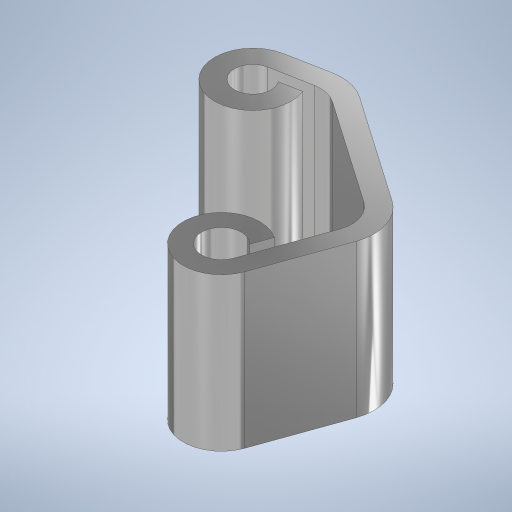
# Autodesk Inventor part: Linkage for inset hinge
Saved by Autodesk Inventor 2024 (Build 280153000, 153)
## iProperties
Created: 2008-03-26
Part Number: Linkage for inset hinge
Document SubType Name: Modeling
Designer: G.K.
Material: Steel
Description: Linkage for inset hinge
Authority: Design by UAB Čeli APS
Mass: 4.02681 g
Surface Area: 9.41342 cm^2
Volume: 0.512969 cm^3
Density: 7.85 g/cm^3
Appearance: Chrome - Polished
Mase: 0.00402681
Autodesk Inventor part; units mm, degrees
ref_plane "YZ Plane" through (0, 0, 0) normal (1, 0, 0) x (0, 1, 0)
ref_plane "XZ Plane" through (0, 0, 0) normal (0, 1, 0) x (-1, 0, 0)
ref_plane "XY Plane" through (0, 0, 0) normal (0, 0, 1) x (1, 0, 0)
sketch "Sketch1" plane through (0, 0, 0) normal (0, 0, 1) x (1, 0, 0)
  arc A0 (10.377, 42.8791) -> (11.579, 42.394) centre (10.6, 41.7) ccw
  arc A1 (10.1355, 44.1565) -> (12.9139, 42.6464) centre (10.6, 41.7) ccw
  arc A2 (20.2623, 33.4501) -> (21.2356, 30.5256) centre (18.8812, 31.3663) ccw
  line L0 (10.1355, 44.1565) -> (14.0658, 44.8997)
  line L1 (14.0658, 44.8997) -> (23.9257, 38.0598)
  line L2 (23.9257, 38.0598) -> (21.2356, 30.5256)
  line L3 (10.377, 42.8791) -> (13.7723, 43.5211)
  line L4 (13.7723, 43.5211) -> (22.4517, 37.5001)
  line L5 (22.4517, 37.5001) -> (20.1055, 30.9291)
  line L6 (11.579, 42.394) -> (12.9139, 42.6464)
  line L7 (20.2623, 33.4501) -> (19.834, 32.2506)
  arc A3 (19.834, 32.2506) -> (20.1055, 30.9291) centre (18.8812, 31.3663) ccw
  line L8 (10.6, 41.7) -> (18.8812, 31.3663) construction
  point P0 (0, 0)
  dimension "d0" = 5
  dimension "d1" = 5
  dimension "d2" = 1.3
  dimension "d5" = 1.3
  dimension "d6" = 12
  dimension "d7" = 4
  dimension "d8" = 8
  dimension "d9" = 0.7
  dimension "d10" = 0.7
  dimension "d11" = 62
  dimension "d12" = 1.2
  constraints: 18 end point, 8 point on circle, 5 parallel, 4 centre point, 4 tangent, 2 coincident, 4 other
  measures "d0" diameter of A1
  measures "d1" diameter of A2
  measures "d2" distance between parallel lines of L1 L4
  measures "d5" distance between parallel lines of L3 L0
  measures "d6" distance of L0.end L1.end
  measures "d7" distance of L0.start L0.end
  measures "d8" distance of L1.end L2.end
  measures "d9" distance between parallel lines of L3 L6
  measures "d10" distance between parallel lines of L5 L7
  measures "d11" angle of L8 L3
  measures "d12" distance between parallel lines of L2 L5
extrude "Extrusion1" add sketch "Sketch1" along normal mid plane 10
fillet "Fillet1" radius 2 2 edges at (22.4517, 37.5001, 0) (13.7723, 43.5211, 0)
fillet "Fillet1" radius 3 2 edges at (14.0658, 44.8997, 0) (23.9257, 38.0598, 0)
body "Solid1"
